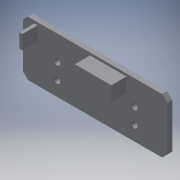
# Autodesk Inventor part: LaserMount
Saved by Autodesk Inventor 2016 (Build 200138000, 138)
## iProperties
Created: 2016-01-27
Part Number: LaserMount
Material: Generic
Document SubType Name: Modeling
Designer: seve
Density: 1 g/cm^3
Appearance: Default
Author: seve
Autodesk Inventor part; units mm, degrees
ref_plane "YZ Plane" through (0, 0, 0) normal (1, 0, 0) x (0, 1, 0)
ref_plane "XZ Plane" through (0, 0, 0) normal (0, 1, 0) x (-1, 0, 0)
ref_plane "XY Plane" through (0, 0, 0) normal (0, 0, 1) x (1, 0, 0)
sketch "Sketch1" plane through (0, 0, 0) normal (0, 0, 1) x (1, 0, 0)
  circle A0 centre (3.75, 22.13) radius 2 projected
  circle A1 centre (3.75, 12.13) radius 2 projected
  circle A2 centre (-44.75, 22.13) radius 2 projected
  circle A3 centre (-44.75, 12.13) radius 2 projected
  line L0 (0, 3) -> (-41, 3) projected
  line L1 (-5.5, 37.5) -> (-35.5, 37.5) projected
  line L2 (24.4262, 37.5) -> (-66.1967, 37.5)
  line L3 (-66.1967, 37.5) -> (-66.1967, 3)
  line L4 (-66.1967, 3) -> (24.4262, 3)
  line L5 (24.4262, 3) -> (24.4262, 37.5)
  point P0 (0, 0)
  constraints: 8 end point, 2 parallel, 1 horizontal, 1 perpendicular
extrude "Extrusion1" add sketch "Sketch1" along normal blind 3.175
chamfer "Chamfer1" distance 3.175 angle 45 4 edges at (-66.1967, 3, 1.5875) (-66.1967, 37.5, 1.5875) (24.4262, 3, 1.5875) (24.4262, 37.5, 1.5875)
sketch "Sketch2" plane through (0, 0, 3.175) normal (0, 0, 1) x (1, 0, 0)
  line L0 (-1.1418, 35.8637) -> (-24.0515, 35.8637)
  line L1 (-24.0515, 35.8637) -> (-24.0515, 26.9046)
  line L2 (-24.0515, 26.9046) -> (-1.1418, 26.9046)
  line L3 (-1.1418, 26.9046) -> (-1.1418, 35.8637)
  line L4 (-56.9442, 35.8637) -> (-58.992, 35.8637)
  line L5 (-58.992, 35.8637) -> (-58.992, 26.9046)
  line L6 (-58.992, 26.9046) -> (-56.9442, 26.9046)
  line L7 (-56.9442, 26.9046) -> (-56.9442, 35.8637)
  point P0 (0, 0)
  constraints: 16 end point, 4 parallel, 2 horizontal, 2 perpendicular
extrude "Extrusion2" add sketch "Sketch2" along normal blind 9.525
body "Solid1"
